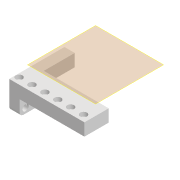
# Autodesk Inventor part: 30_cellSTORM_UC2_Laser_slider
Saved by Autodesk Inventor 2022 (Build 260153000, 153)
## iProperties
Created: 2021-11-15
Part Number: 30_cellSTORM_UC2_Laser_slider
Material: Generic
Document SubType Name: Modeling
Designer: diederichbenedict
Density: 1 g/cm^3
Appearance: Default
Author: diederichbenedict
Autodesk Inventor part; units mm, degrees
ref_plane "YZ Plane" through (0, 0, 0) normal (1, 0, 0) x (0, 1, 0)
ref_plane "XZ Plane" through (0, 0, 0) normal (0, 1, 0) x (-1, 0, 0)
ref_plane "XY Plane" through (0, 0, 0) normal (0, 0, 1) x (1, 0, 0)
ref_plane "Work Plane1" through (18, 18.5, -30) normal (0, 1, 0) x (0, 0, -1)
sketch "Sketch1" plane through (18, 18.5, -30) normal (0, 1, 0) x (0, 0, -1)
  line L0 (-30.1565, -29.8905) -> (-15.0465, -29.8905) construction
  line L1 (-30, -38) -> (-30, 18) construction
  circle A0 centre (-25, -20) radius 1.45 construction
  circle A1 centre (25, -20) radius 1.45 construction
  circle A2 centre (25, 0) radius 1.45 construction
  circle A3 centre (-25, 0) radius 1.45 construction
  circle A4 centre (10, -35) radius 1.45 construction
  circle A5 centre (10, 15) radius 1.45 construction
  circle A6 centre (-10, 15) radius 1.45 construction
  circle A7 centre (-10, -35) radius 1.45 construction
  circle A8 centre (25, 15) radius 2.325 construction
  circle A9 centre (-25, -35) radius 2.325 construction
  circle A10 centre (25, -35) radius 2.325 construction
  circle A11 centre (-25, 15) radius 2.325 construction
  line L2 (-28, 20) -> (-30, 18) construction
  line L3 (-28, 20) -> (28, 20) construction
  line L4 (30, 18) -> (28, 20) construction
  line L5 (30, 18) -> (30, -38) construction
  line L6 (28, -40) -> (30, -38) construction
  line L7 (28, -40) -> (-28, -40) construction
  line L8 (-30, -38) -> (-28, -40) construction
  line L9 (-30, -38) -> (-30, 18) construction
  circle A12 centre (17.5, -27.5) radius 1.95 construction
  circle A13 centre (-17.5, 7.5) radius 1.95 construction
  circle A14 centre (-17.5, -27.5) radius 1.95 construction
  circle A15 centre (17.5, 7.5) radius 1.95 construction
  circle A16 centre (0, -10) radius 7.5 construction
  line L10 (-0.1565, 20) -> (-30.1565, 20)
  line L11 (-30.1565, 20) -> (-30.1565, 30)
  line L12 (-30.1565, 30) -> (-0.1565, 30)
  line L13 (-0.1565, 30) -> (-0.1565, 20)
  line L14 (-30.1565, 30) -> (-53.7065, 30)
  line L15 (-53.7065, 30) -> (-53.7065, -42.9244)
  line L16 (-53.7065, -42.9244) -> (-30.1565, -42.9244)
  line L17 (-30.1565, -42.9244) -> (-30.1565, 30)
  circle A17 centre (-47.5565, 1.5545) radius 1.75 construction
  circle A18 centre (-47.5565, -10.9455) radius 1.75 construction
  circle A19 centre (-47.5565, -23.4455) radius 1.75 construction
  circle A20 centre (-47.5565, -35.9455) radius 1.75 construction
  line L18 (-41.6065, -40.3471) -> (-53.7065, -40.3471) construction
  line L19 (-41.6065, -40.3471) -> (-41.6065, 9.6529) construction
  line L20 (-41.6065, 9.6529) -> (-53.7065, 9.6529) construction
  line L21 (-53.7065, -40.3471) -> (-53.7065, 9.6529) construction
  circle A21 centre (-47.5565, -48.4455) radius 1.75 construction
  circle A22 centre (-47.5565, -60.9455) radius 1.75 construction
  circle A23 centre (-47.5565, -73.4455) radius 1.75 construction
  circle A24 centre (-47.5565, -85.9455) radius 1.75 construction
  line L22 (-41.6065, -90.3471) -> (-53.7065, -90.3471) construction
  line L23 (-41.6065, -90.3471) -> (-41.6065, -40.3471) construction
  line L24 (-41.6065, -40.3471) -> (-53.7065, -40.3471) construction
  line L25 (-53.7065, -90.3471) -> (-53.7065, -40.3471) construction
  point P0 (-30.1565, 20)
  dimension "d0" = 10
  dimension "d1" = 30
  constraints: 16 end point, 4 parallel, 2 horizontal, 2 perpendicular, 2 point on line
  measures "d0" distance of L10.end L11.end
  measures "d1" distance between parallel lines of L11 L13
extrude "Extrusion1" add sketch "Sketch1" against normal blind 12
sketch "Sketch2" plane through (18, 18.5, -30) normal (0, 1, 0) x (1, 0, 0)
  circle A0 centre (35.9455, -47.5565) radius 1.75 projected
  point P0 (-18, -30)
hole "Hole1" at (53.9455, 18.5, 17.5565) direction (0, -1, 0) diameter 2.8 end through all counterbore diameter 6.5 counterbore depth 4
pattern_linear "Rectangular Pattern1" count 9 spacing 12.5 along (-1, 0, 0) of "Hole1"
sketch "Sketch3" plane through (18, 6.5, -30) normal (0, -1, 0) x (1, 0, 0)
  line L0 (-30, 53.7065) -> (-30, 0.1565) projected
  line L1 (-30, 0.1565) -> (-20, 0.1565) projected
  line L2 (-20, 0.1565) -> (-20, 30.1565) projected
  line L3 (-20, 30.1565) -> (42.9244, 30.1565) projected
  line L4 (42.9244, 30.1565) -> (42.9244, 53.7065) projected
  line L5 (42.9244, 53.7065) -> (-30, 53.7065) projected
  line L6 (-30, 53.7065) -> (42.9244, 53.7065) projected
  line L7 (-30, 53.7065) -> (-20, 53.7065)
  line L8 (-20, 53.7065) -> (-20, 29.1031)
  line L9 (-20, 29.1031) -> (-30, 29.1031)
  line L10 (-30, 29.1031) -> (-30, 53.7065)
  point P0 (-18, 30)
  point P1 (-30, 29.1031)
  dimension "d14" = 10
  constraints: 8 end point, 2 parallel, 1 horizontal, 1 perpendicular
  measures "d14" distance of L8.end L9.end
extrude "Extrusion2" add sketch "Sketch3" along normal blind 15 contours L5 L8 L2 L9 L0
sketch "Sketch4" plane through (-12, 18.5, -29.8435) normal (-1, 0, 0) x (0, 0, 1)
  line L0 (0, 0) -> (53.55, 0) projected
  line L1 (0, 0) -> (0, -12) projected
  line L2 (28.9466, -12) -> (0, -12) projected
  line L3 (28.9466, -12) -> (28.9466, -27) projected
  line L4 (53.55, -27) -> (28.9466, -27) projected
  line L5 (53.55, 0) -> (53.55, -27) projected
  circle A0 centre (40.6, -17.5571) radius 2.1 projected
  circle A1 centre (47.6565, -22.005) radius 1.6829
  arc A2 (53.5014, -16.3734) -> (53.6565, -16.1421) centre (53.4065, -16.1421) ccw construction
  arc A3 (53.5014, -16.3734) -> (52.9237, -16.8727) centre (53.9565, -17.4838) ccw construction
  arc A4 (52.7304, -16.9945) -> (52.9237, -16.8727) centre (52.7086, -16.7455) ccw construction
  line L6 (52.7304, -16.9945) -> (52.3847, -17.0247) construction
  arc A5 (52.3847, -17.0247) -> (52.1565, -17.2738) centre (52.4065, -17.2738) ccw construction
  line L7 (52.1565, -17.2738) -> (52.1565, -17.7262) construction
  arc A6 (52.1565, -17.7262) -> (52.3847, -17.9753) centre (52.4065, -17.7262) ccw construction
  line L8 (52.3847, -17.9753) -> (52.7513, -18.0073) construction
  arc A7 (52.9411, -18.1232) -> (52.7513, -18.0073) centre (52.7295, -18.2564) ccw construction
  arc A8 (52.9411, -18.1232) -> (53.5014, -18.5941) centre (53.9565, -17.4838) ccw construction
  arc A9 (53.6565, -18.8254) -> (53.5014, -18.5941) centre (53.4065, -18.8254) ccw construction
  line L9 (53.6565, -18.8254) -> (53.6565, -19.5) construction
  line L10 (53.6565, -19.5) -> (53.1565, -20) construction
  line L11 (53.1565, -20) -> (42.1566, -20) construction
  line L12 (42.1566, -20) -> (41.6566, -19.5) construction
  line L13 (41.6566, -19.5) -> (41.6566, -18.8254) construction
  arc A10 (41.8117, -18.5941) -> (41.6566, -18.8254) centre (41.9066, -18.8254) ccw construction
  arc A11 (41.8117, -18.5941) -> (42.372, -18.1232) centre (41.3566, -17.4838) ccw construction
  arc A12 (42.5618, -18.0073) -> (42.372, -18.1232) centre (42.5836, -18.2564) ccw construction
  line L14 (42.5618, -18.0073) -> (42.9283, -17.9753) construction
  arc A13 (42.9283, -17.9753) -> (43.1566, -17.7262) centre (42.9066, -17.7262) ccw construction
  line L15 (43.1566, -17.7262) -> (43.1566, -17.2738) construction
  arc A14 (43.1566, -17.2738) -> (42.9283, -17.0247) centre (42.9066, -17.2738) ccw construction
  line L16 (42.9283, -17.0247) -> (42.5827, -16.9945) construction
  arc A15 (42.3894, -16.8727) -> (42.5827, -16.9945) centre (42.6045, -16.7455) ccw construction
  arc A16 (42.3894, -16.8727) -> (41.8117, -16.3734) centre (41.3566, -17.4838) ccw construction
  arc A17 (41.6566, -16.1421) -> (41.8117, -16.3734) centre (41.9066, -16.1421) ccw construction
  line L17 (41.6566, -16.1421) -> (41.6566, -15) construction
  line L18 (41.6566, -15) -> (35.0566, -15) construction
  line L19 (35.0566, -15) -> (34.4566, -15.6) construction
  line L20 (34.4566, -15.6) -> (34.4566, -23.4) construction
  line L21 (34.4566, -23.4) -> (35.6565, -24.6) construction
  line L22 (35.6565, -24.6) -> (59.6565, -24.6) construction
  line L23 (59.6565, -24.6) -> (60.8565, -23.4) construction
  line L24 (60.8565, -23.4) -> (60.8565, -15.6) construction
  line L25 (60.8565, -15.6) -> (60.2565, -15) construction
  line L26 (60.2565, -15) -> (53.6565, -15) construction
  line L27 (53.6565, -15) -> (53.6565, -16.1421) construction
  circle A18 centre (40.7565, -22.005) radius 2.1 construction
  circle A19 centre (54.5565, -22.005) radius 2.1 construction
  point P0 (29.8435, -18.5)
  constraints: 1 centre point
hole "Hole2" at (-12, -3.505, 17.8131) direction (1, 0, 0) diameter 6.1 end through all
fillet "Fillet1" radius 4 3 edges at (-7, -8.5, 23.7065) (-7, -8.5, -0.8969) (-7, 6.5, -0.8969)
sketch "Sketch5" plane through (18, -8.5, -30) normal (0, -1, 0) x (1, 0, 0)
  line L0 (-20, 43.8065) -> (-30, 43.8065) construction
  circle A0 centre (-22.4542, 43.5587) radius 1.4
  circle A1 centre (-27.2211, 43.5587) radius 1.4
  line L1 (-20, 44.7631) -> (-30, 44.7631) projected
  point P0 (-18, 30)
  dimension "d28" = 2.8
  dimension "d29" = 2.8
  constraints: 2 centre point
  measures "d28" diameter of A0
  measures "d29" diameter of A1
extrude "Extrusion3" cut sketch "Sketch5" against normal blind 15
body "Solid1"
